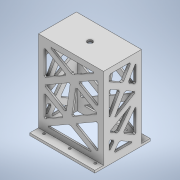
# Autodesk Inventor part: Shroud
Saved by Autodesk Inventor 2020 (Build 240168000, 168)
## iProperties
Created: 2019-08-01
Part Number: Shroud
Material: Generic
Document SubType Name: Modeling
Designer: Alex
Density: 1 g/cm^3
Appearance: Default
Author: Alex
Autodesk Inventor part; units mm, degrees
ref_plane "YZ Plane" through (0, 0, 0) normal (1, 0, 0) x (0, 1, 0)
ref_plane "XZ Plane" through (0, 0, 0) normal (0, 1, 0) x (-1, 0, 0)
ref_plane "XY Plane" through (0, 0, 0) normal (0, 0, 1) x (1, 0, 0)
sketch "Sketch3" plane through (0, 0, 0) normal (0, 1, 0) x (-1, 0, 0)
  line L0 (41.166, -35) -> (-41.166, -35)
  line L1 (-41.166, -35) -> (-41.166, 35)
  line L2 (-41.166, 35) -> (41.166, 35)
  line L3 (41.166, 35) -> (41.166, -35)
  line L4 (38.166, -22) -> (-38.166, -22)
  line L5 (-38.166, -22) -> (-38.166, 22)
  line L6 (-38.166, 22) -> (38.166, 22)
  line L7 (38.166, 22) -> (38.166, -22)
  point P0 (0, 0)
  point P1 (0, -35)
  point P2 (41.166, 0)
  point P3 (-38.166, 0)
  point P4 (0, -22)
  dimension "d7" = 82.332
  dimension "d8" = 70
  dimension "d10" = 13
  dimension "d12" = 3
  constraints: 16 end point, 4 midpoint, 4 parallel, 2 horizontal, 2 horizontal alignment, 2 perpendicular, 2 vertical alignment
  measures "d7" distance of L1.end L2.end
  measures "d8" distance of L0.end L1.end
  measures "d10" distance between parallel lines of L0 L4
  measures "d12" distance between parallel lines of L1 L5
extrude "Extrusion2" add sketch "Sketch3" along normal blind 3
sketch "Sketch4" plane through (0, 3, 0) normal (0, 1, 0) x (1, 0, 0)
  line L0 (41.166, -35) -> (41.166, 35) construction
  line L1 (41.166, 35) -> (-41.166, 35) construction
  line L2 (-41.166, 35) -> (-41.166, -35) construction
  line L3 (-41.166, -35) -> (41.166, -35) construction
  line L4 (38.166, -22) -> (-38.166, -22) construction
  line L5 (-38.166, -22) -> (-38.166, 22) construction
  line L6 (-38.166, 22) -> (38.166, 22) construction
  line L7 (38.166, 22) -> (38.166, -22) construction
  line L8 (-41.166, 35) -> (-41.166, -35) construction
  line L9 (-41.166, 24) -> (-41.166, -24)
  line L10 (41.166, -24) -> (-41.166, -24)
  line L11 (41.166, -24) -> (41.166, 24)
  line L12 (41.166, -35) -> (41.166, 35) construction
  line L13 (-41.166, 24) -> (41.166, 24)
  line L14 (-38.166, 22) -> (38.166, 22) projected
  line L15 (-38.166, -22) -> (38.166, -22)
  line L16 (38.166, -22) -> (38.166, 22)
  line L17 (38.166, 22) -> (-38.166, 22)
  line L18 (-38.166, 22) -> (-38.166, -22)
  point P0 (0, 0)
  point P1 (-41.166, 0)
  point P2 (-38.166, 0)
  dimension "d16" = 2
  constraints: 16 end point, 4 point on line, 2 horizontal, 2 midpoint, 2 parallel, 2 perpendicular, 1 horizontal alignment
  measures "d16" distance between parallel lines of L13 L6
extrude "Extrusion3" add sketch "Sketch4" along normal blind 100
sketch "Sketch5" plane through (0, 103, 0) normal (0, 1, 0) x (1, 0, 0)
  line L0 (-41.166, -24) -> (41.166, -24) projected
  line L1 (41.166, -24) -> (41.166, 24) projected
  line L2 (41.166, 24) -> (-41.166, 24) projected
  line L3 (-41.166, 24) -> (-41.166, -24) projected
  line L4 (38.166, 22) -> (38.166, -22) construction
  line L5 (38.166, -22) -> (-38.166, -22) construction
  line L6 (-38.166, -22) -> (-38.166, 22) construction
  line L7 (-38.166, 22) -> (38.166, 22) construction
  point P0 (0, 0)
extrude "Extrusion4" add sketch "Sketch5" along normal blind 3
sketch "Sketch6" plane through (-41.166, 0, -35) normal (-1, 0, 0) x (0, 0, 1)
  line L0 (0, 0) -> (70, 0) construction
  line L1 (57, 0) -> (13, 0) construction
  arc A0 (39, 0) -> (31, 0) centre (35, 0) ccw
  line L2 (31, 0) -> (39, 0)
  point P0 (35, 0)
  dimension "d22" = 4
  constraints: 2 end point, 2 point on circle, 2 point on line, 1 centre point, 1 coincident, 1 midpoint
  measures "d22" radius of A0
extrude "Extrusion5" cut sketch "Sketch6" against normal up to surface (3 mm away)
sketch "Sketch7" plane through (0, 3, 0) normal (0, 1, 0) x (1, 0, 0)
  line L0 (41.166, -35) -> (41.166, 35) construction
  line L1 (41.166, 35) -> (-41.166, 35) construction
  line L2 (-41.166, -35) -> (41.166, -35) construction
  point P0 (0, 0)
  point P1 (33.834, 27)
  point P2 (1.334, 27)
  point P3 (-31.166, 27)
  point P4 (-31.166, -27)
  point P5 (1.334, -27)
  point P6 (33.834, -27)
  dimension "d25" = 7.332
  dimension "d26" = 39.832
  dimension "d27" = 72.332
  dimension "d28" = 8
  dimension "d29" = 8
  constraints: 4 horizontal alignment, 3 vertical alignment
  measures "d25" distance from line of point (33.834, 27) L0
  measures "d26" distance from line of point (1.334, 27) L0
  measures "d27" distance from line of point (-31.166, 27) L0
  measures "d28" distance from line of L1 point (33.834, 27)
  measures "d29" distance from line of L2 point (33.834, -27)
hole "Hole1" at (33.834, 3, -27) at (1.334, 3, -27) at (-31.166, 3, -27) at (-31.166, 3, 27) at (1.334, 3, 27) at (33.834, 3, 27) direction (0, -1, 0) diameter 3 end through all
sketch "Sketch8" plane through (-41.166, 3, 24) normal (0, 0, 1) x (1, 0, 0)
  line L0 (82.332, 0) -> (0, 0) construction
  line L1 (82.332, 0) -> (82.332, 103) construction
  line L2 (0, 103) -> (82.332, 103) construction
  line L3 (0, 0) -> (0, 103) construction
  line L4 (75.332, 96) -> (75.332, 7) construction
  line L5 (75.332, 7) -> (7, 7) construction
  line L6 (7, 7) -> (7, 96) construction
  line L7 (7, 96) -> (75.332, 96) construction
  line L8 (14.0115, 96) -> (75.332, 60.5966) construction
  line L9 (75.332, 52.5137) -> (7, 91.9652) construction
  line L10 (75.332, 52.5137) -> (7, 13.0622) construction
  line L11 (10.5, 7) -> (75.332, 44.4308) construction
  line L12 (7, 13.0622) -> (10.5, 7) construction
  line L13 (35.9217, 75.2672) -> (7, 58.5692) construction
  line L14 (7, 50.4863) -> (42.9217, 71.2257) construction
  line L15 (7, 50.4863) -> (39.4103, 31.7743) construction
  line L16 (7, 42.4034) -> (32.4103, 27.7328) construction
  line L17 (42.9217, 79.3087) -> (71.832, 96) construction
  line L18 (75.332, 89.9378) -> (49.9217, 75.2672) construction
  line L19 (71.832, 96) -> (75.332, 89.9378) construction
  line L20 (39.4103, 23.6913) -> (75.332, 2.9519) construction
  line L21 (46.4103, 27.7328) -> (75.332, 11.0348) construction
  line L22 (40.3575, 69.7453) -> (35.0516, 34.2907) construction
  line L23 (47.2804, 68.7093) -> (41.9745, 33.2547) construction
  line L24 (40.3575, 69.7453) -> (47.2804, 68.7093) construction
  line L25 (35.0516, 34.2907) -> (41.9745, 33.2547) construction
  line L26 (15.7435, 95) -> (41.1897, 80.3087)
  line L27 (44.6538, 80.3087) -> (70.0999, 95)
  line L28 (69.832, 96) -> (16.0115, 96)
  line L29 (34.1897, 76.2672) -> (8.7321, 90.9652)
  line L30 (7, 60.5692) -> (7, 89.9652)
  line L31 (8.7321, 59.5692) -> (34.1897, 74.2672)
  line L32 (51.6538, 76.2672) -> (73.5999, 88.9378)
  line L33 (75.332, 62.5966) -> (75.332, 87.9378)
  line L34 (51.6538, 74.2672) -> (73.5999, 61.5966)
  line L35 (46.9844, 66.7313) -> (42.2705, 35.2327)
  line L36 (43.7065, 34.2547) -> (73.5999, 51.5137)
  line L37 (73.5999, 53.5137) -> (49.0125, 67.7093)
  line L38 (8.7321, 49.4863) -> (33.3195, 35.2907)
  line L39 (35.3476, 36.2687) -> (40.0615, 67.7673)
  line L40 (8.7321, 51.4863) -> (38.6255, 68.7453)
  line L41 (7, 40.4034) -> (7, 15.0622)
  line L42 (8.7321, 14.0622) -> (30.6782, 26.7328)
  line L43 (30.6782, 28.7328) -> (8.7321, 41.4034)
  line L44 (12.2321, 8) -> (37.6782, 22.6913)
  line L45 (41.1423, 22.6913) -> (66.5885, 8)
  line L46 (66.3205, 7) -> (12.5, 7)
  line L47 (48.1423, 28.7328) -> (73.5999, 43.4308)
  line L48 (75.332, 42.4308) -> (75.332, 13.0348)
  line L49 (48.1423, 26.7328) -> (73.5999, 12.0348)
  line L50 (8.7321, 90.9652) -> (7, 89.9652)
  line L51 (7, 60.5692) -> (8.7321, 59.5692)
  line L52 (7, 60.5692) -> (8.7321, 59.5692)
  line L53 (34.1897, 74.2672) -> (34.1897, 76.2672)
  line L54 (15.7435, 95) -> (16.0115, 96)
  line L55 (70.0999, 95) -> (69.832, 96)
  line L56 (69.832, 96) -> (70.0999, 95)
  line L57 (41.1897, 80.3087) -> (44.6538, 80.3087)
  line L58 (51.6538, 74.2672) -> (51.6538, 76.2672)
  line L59 (73.5999, 88.9378) -> (75.332, 87.9378)
  line L60 (73.5999, 61.5966) -> (75.332, 62.5966)
  line L61 (49.0125, 67.7093) -> (46.9844, 66.7313)
  line L62 (42.2705, 35.2327) -> (43.7065, 34.2547)
  line L63 (73.5999, 53.5137) -> (73.5999, 51.5137)
  line L64 (8.7321, 41.4034) -> (7, 40.4034)
  line L65 (8.7321, 41.4034) -> (7, 40.4034)
  line L66 (8.7321, 14.0622) -> (7, 15.0622)
  line L67 (30.6782, 26.7328) -> (30.6782, 28.7328)
  line L68 (12.2321, 8) -> (12.5, 7)
  line L69 (66.5885, 8) -> (66.3205, 7)
  line L70 (37.6782, 22.6913) -> (41.1423, 22.6913)
  line L71 (48.1423, 28.7328) -> (48.1423, 26.7328)
  line L72 (73.5999, 43.4308) -> (75.332, 42.4308)
  line L73 (73.5999, 12.0348) -> (75.332, 13.0348)
  line L74 (8.7321, 49.4863) -> (8.7321, 51.4863)
  line L75 (8.7321, 49.4863) -> (8.7321, 51.4863)
  line L76 (38.6255, 68.7453) -> (40.0615, 67.7673)
  line L77 (33.3195, 35.2907) -> (35.3476, 36.2687)
  point P0 (41.166, -3)
  point P1 (68.3205, 7)
  dimension "d37" = 7
  dimension "d38" = 30
  dimension "d39" = 60
  dimension "d40" = 7
  dimension "d41" = 7
  dimension "d42" = 7
  dimension "d43" = 7
  dimension "d44" = 60
  dimension "d45" = 60
  dimension "d46" = 7
  dimension "d49" = 2
  dimension "d50" = 2
  dimension "d51" = 2
  dimension "d52" = 2
  dimension "d53" = 2
  dimension "d54" = 2
  dimension "d55" = 2
  dimension "d56" = 2
  dimension "d57" = 2
  dimension "d58" = 2
  dimension "d59" = 2
  dimension "d60" = 2
  dimension "d61" = 2
  dimension "d62" = 2
  dimension "d63" = 2
  dimension "d64" = 2
  dimension "d65" = 2
  dimension "d66" = 2
  dimension "d67" = 2
  dimension "d68" = 2
  dimension "d69" = 2
  dimension "d70" = 2
  dimension "d71" = 2
  dimension "d72" = 2
  dimension "d73" = 2
  dimension "d74" = 2
  dimension "d75" = 2
  dimension "d76" = 2
  dimension "d77" = 2
  dimension "d78" = 2
  dimension "d79" = 2
  dimension "d80" = 2
  dimension "d81" = 2
  dimension "d82" = 2
  dimension "d83" = 2
  dimension "d84" = 2
  dimension "d85" = 2
  dimension "d86" = 2
  dimension "d87" = 2
  dimension "d88" = 2
  dimension "d89" = 2
  dimension "d90" = 2
  dimension "d91" = 2
  dimension "d92" = 2
  dimension "d93" = 2
  dimension "d94" = 2
  dimension "d95" = 2
  dimension "d96" = 2
  dimension "d97" = 2
  dimension "d98" = 2
  dimension "d99" = 2
  dimension "d100" = 2
  dimension "d101" = 2
  dimension "d102" = 2
  constraints: 148 end point, 91 point on line, 20 collinear, 9 parallel, 7 perpendicular, 3 other
  measures "d37" distance between parallel lines of L2 L7
  measures "d38" angle of L11 L5
  measures "d39" angle of L10 L9
  measures "d40" distance between parallel lines of L11 L10
  measures "d41" distance between parallel lines of L8 L9
  measures "d42" distance between parallel lines of L13 L14
  measures "d43" distance between parallel lines of L15 L16
  measures "d44" angle of L10 L16
  measures "d45" angle of L14 L15
  measures "d46" distance between parallel lines of L23 L22
  measures "d49" distance of L29.end L9.end
  measures "d50" distance of L30.end L9.end
  measures "d51" distance of L51.start L13.end
  measures "d52" distance of L51.end L13.end
  measures "d53" distance of L30.start point (7, 58.569)
  measures "d54" distance of L31.start point (7, 58.569)
  measures "d55" distance of L31.end L13.start
  measures "d56" distance of L29.start L13.start
  measures "d57" distance of L26.start L8.start
  measures "d58" distance of L28.end L8.start
  measures "d59" distance of L55.start L17.end
  measures "d60" distance of L55.end L17.end
  measures "d61" distance of L28.start point (71.832, 96)
  measures "d62" distance of L27.end point (71.832, 96)
  measures "d63" distance of L26.end L17.start
  measures "d64" distance of L27.start L17.start
  measures "d65" distance of L34.start L18.end
  measures "d66" distance of L32.start L18.end
  measures "d67" distance of L32.end L18.start
  measures "d68" distance of L33.end L18.start
  measures "d69" distance of L34.end L8.end
  measures "d70" distance of L33.start L8.end
  measures "d71" distance of L37.end L23.start
  measures "d72" distance of L35.start L23.start
  measures "d73" distance of L35.end L23.end
  measures "d74" distance of L36.start L23.end
  measures "d75" distance of L37.start L9.start
  measures "d76" distance of L36.end L9.start
  measures "d77" distance of L64.start L16.start
  measures "d78" distance of L64.end L16.start
  measures "d79" distance of L43.end point (7, 42.403)
  measures "d80" distance of L41.start point (7, 42.403)
  measures "d81" distance of L42.start L10.end
  measures "d82" distance of L41.end L10.end
  measures "d83" distance of L42.end L16.end
  measures "d84" distance of L43.start L16.end
  measures "d85" distance of L44.start L11.start
  measures "d86" distance of L46.end L11.start
  measures "d87" distance of L45.end point (68.321, 7)
  measures "d88" distance of L46.start point (68.321, 7)
  measures "d89" distance of L44.end L20.start
  measures "d90" distance of L45.start L20.start
  measures "d91" distance of L47.start L21.start
  measures "d92" distance of L49.start L21.start
  measures "d93" distance of L47.end L11.end
  measures "d94" distance of L48.start L11.end
  measures "d95" distance of L49.end L21.end
  measures "d96" distance of L48.end L21.end
  measures "d97" distance of L74.start L14.start
  measures "d98" distance of L74.end L14.start
  measures "d99" distance of L38.start point (7, 50.486)
  measures "d100" distance of L40.start point (7, 50.486)
  measures "d101" distance of L40.end L22.start
  measures "d102" distance of L39.end L22.start
extrude "Extrusion6" cut sketch "Sketch8" against normal through all
sketch "Sketch9" plane through (-41.166, 3, 24) normal (-1, 0, 0) x (0, 0, 1)
  arc A0 (-20, -3) -> (-28, -3) centre (-24, -3) ccw construction
  line L0 (-20, -3) -> (11, -3) construction
  line L1 (11, -3) -> (11, 0) construction
  line L2 (0, 0) -> (11, 0) construction
  line L3 (0, 0) -> (0, 103) construction
  line L4 (-48, 103) -> (0, 103) construction
  line L5 (-48, 0) -> (-48, 103) construction
  line L6 (-59, 0) -> (-48, 0) construction
  line L7 (-59, -3) -> (-59, 0) construction
  line L8 (-59, -3) -> (-28, -3) construction
  line L9 (-41, 96) -> (-7, 96) construction
  line L10 (-7, 96) -> (-7, 7) construction
  line L11 (-7, 7) -> (-41, 7) construction
  line L12 (-41, 7) -> (-41, 96) construction
  line L13 (-41, 13.0622) -> (-7, 32.6921) construction
  line L14 (-37.5, 7) -> (-7, 24.6092) construction
  line L15 (-7, 32.6921) -> (-41, 52.322) construction
  line L16 (-7, 88.1177) -> (-41, 68.4878) construction
  line L17 (-41, 60.4049) -> (-7, 40.775) construction
  line L18 (-41, 60.4049) -> (-7, 80.0348) construction
  line L19 (-41, 92.5) -> (-30.6024, 74.4909) construction
  line L20 (-24.5402, 77.9909) -> (-34.9378, 96) construction
  line L21 (-41, 92.5) -> (-34.9378, 96) construction
  line L22 (-41, 13.0622) -> (-37.5, 7) construction
  line L23 (-27.1024, 68.4287) -> (-13.2048, 44.3573) construction
  line L24 (-21.0402, 71.9287) -> (-7, 47.6103) construction
  line L25 (-12.6013, 7) -> (-41, 44.8898) construction
  line L26 (-7, 11.1982) -> (-35.3987, 49.0881) construction
  line L27 (-12.6013, 7) -> (-7, 11.1982) construction
  line L28 (-41, 44.8898) -> (-35.3987, 49.0881) construction
  line L29 (-33.9378, 94.2679) -> (-25.5402, 79.7229)
  line L30 (-22.8082, 78.9909) -> (-7, 88.1177)
  line L31 (-7, 88.1177) -> (-7, 94)
  line L32 (-9, 96) -> (-32.9378, 96)
  line L33 (-40, 90.7679) -> (-31.6024, 76.2229)
  line L34 (-32.3345, 73.4909) -> (-39.2679, 69.4878)
  line L35 (-41, 90.5) -> (-41, 70.4878)
  line L36 (-19.3082, 72.9287) -> (-8.7321, 79.0348)
  line L37 (-20.0402, 70.1966) -> (-8, 49.3423)
  line L38 (-7, 49.6103) -> (-7, 78.0348)
  line L39 (-26.1024, 66.6966) -> (-14.2048, 46.0894)
  line L40 (-39.2679, 61.4049) -> (-28.8345, 67.4287)
  line L41 (-39.2679, 59.4049) -> (-14.9369, 45.3573)
  line L42 (-34.1992, 47.4877) -> (-19.4436, 27.8007)
  line L43 (-8.7321, 31.6921) -> (-16.5121, 27.2003)
  line L44 (-33.6666, 48.0881) -> (-8.7321, 33.6921)
  line L45 (-39.8005, 43.2895) -> (-25.5494, 24.2755)
  line L46 (-26.082, 21.6751) -> (-39.2679, 14.0622)
  line L47 (-41, 15.0622) -> (-41, 42.8898)
  line L48 (-35.7679, 8) -> (-21.8535, 16.0335)
  line L49 (-13.8008, 8.6004) -> (-18.922, 15.4331)
  line L50 (-14.6013, 7) -> (-35.5, 7)
  line L51 (-8.1995, 12.7986) -> (-12.8162, 18.9583)
  line L52 (-8.7321, 23.6092) -> (-12.2837, 21.5587)
  line L53 (-7, 22.6092) -> (-7, 13.1982)
  line L54 (-41, 70.4878) -> (-39.2679, 69.4878)
  line L55 (-32.3345, 73.4909) -> (-31.6024, 76.2229)
  line L56 (-41, 90.5) -> (-40, 90.7679)
  line L57 (-33.9378, 94.2679) -> (-32.9378, 96)
  line L58 (-22.8082, 78.9909) -> (-25.5402, 79.7229)
  line L59 (-9, 96) -> (-7, 94)
  line L60 (-20.0402, 70.1966) -> (-19.3082, 72.9287)
  line L61 (-7, 78.0348) -> (-8.7321, 79.0348)
  line L62 (-8, 49.3423) -> (-7, 49.6103)
  line L63 (-14.2048, 46.0894) -> (-14.9369, 45.3573)
  line L64 (-39.2679, 59.4049) -> (-39.2679, 61.4049)
  line L65 (-28.8345, 67.4287) -> (-26.1024, 66.6966)
  line L66 (-34.1992, 47.4877) -> (-33.6666, 48.0881)
  line L67 (-19.4436, 27.8007) -> (-16.5121, 27.2003)
  line L68 (-8.7321, 33.6921) -> (-8.7321, 31.6921)
  line L69 (-41, 42.8898) -> (-39.8005, 43.2895)
  line L70 (-41, 15.0622) -> (-39.2679, 14.0622)
  line L71 (-26.082, 21.6751) -> (-25.5494, 24.2755)
  line L72 (-35.7679, 8) -> (-35.5, 7)
  line L73 (-21.8535, 16.0335) -> (-18.922, 15.4331)
  line L74 (-14.6013, 7) -> (-13.8008, 8.6004)
  line L75 (-12.8162, 18.9583) -> (-12.2837, 21.5587)
  line L76 (-8.7321, 23.6092) -> (-7, 22.6092)
  line L77 (-8.1995, 12.7986) -> (-7, 13.1982)
  point P0 (-24, -3)
  point P1 (-18.2441, 26.2003)
  point P2 (-24.3499, 22.6751)
  point P3 (-20.1215, 17.0335)
  point P4 (-14.0157, 20.5587)
  dimension "d105" = 7
  dimension "d106" = 7
  dimension "d107" = 7
  dimension "d108" = 7
  dimension "d109" = 30
  dimension "d110" = 60
  dimension "d111" = 7
  dimension "d112" = 7
  dimension "d113" = 7
  dimension "d114" = 60
  dimension "d115" = 7
  dimension "d116" = 7
  dimension "d117" = 2
  dimension "d118" = 2
  dimension "d119" = 2
  dimension "d120" = 2
  dimension "d121" = 2
  dimension "d122" = 2
  dimension "d123" = 2
  dimension "d124" = 2
  dimension "d125" = 2
  dimension "d126" = 2
  dimension "d127" = 2
  dimension "d128" = 2
  dimension "d129" = 2
  dimension "d130" = 2
  dimension "d131" = 2
  dimension "d132" = 2
  dimension "d133" = 2
  dimension "d134" = 2
  dimension "d135" = 2
  dimension "d136" = 2
  dimension "d137" = 2
  dimension "d138" = 2
  dimension "d139" = 2
  dimension "d140" = 2
  dimension "d141" = 2
  dimension "d142" = 2
  dimension "d143" = 2
  dimension "d144" = 2
  dimension "d145" = 2
  dimension "d146" = 2
  dimension "d147" = 2
  dimension "d148" = 2
  dimension "d149" = 2
  dimension "d150" = 2
  dimension "d151" = 2
  dimension "d152" = 2
  dimension "d153" = 2
  dimension "d154" = 2
  dimension "d155" = 2
  dimension "d156" = 2
  dimension "d157" = 2
  dimension "d158" = 2
  dimension "d159" = 2
  dimension "d160" = 2
  dimension "d161" = 2
  dimension "d162" = 2
  dimension "d163" = 2
  dimension "d164" = 2
  constraints: 136 end point, 79 point on line, 9 collinear, 9 perpendicular, 7 parallel, 3 vertical, 2 horizontal, 10 other
  measures "d105" distance between parallel lines of L5 L12
  measures "d106" distance between parallel lines of L4 L9
  measures "d108" distance from line of L11 L5.start
  measures "d109" angle of L11 L14
  measures "d110" angle of L15 L13
  measures "d111" distance between parallel lines of L14 L13
  measures "d112" distance between parallel lines of L15 L17
  measures "d113" distance between parallel lines of L18 L16
  measures "d114" angle of L18 L17
  measures "d115" distance between parallel lines of L20 L19
  measures "d116" distance between parallel lines of L26 L25
  measures "d117" distance of L35.end L16.end
  measures "d118" distance of L34.end L16.end
  measures "d119" distance of L34.start L19.end
  measures "d120" distance of L33.end L19.end
  measures "d121" distance of L35.start L19.start
  measures "d122" distance of L33.start L19.start
  measures "d123" distance of L29.start L20.end
  measures "d124" distance of L32.end L20.end
  measures "d125" distance of L30.start L20.start
  measures "d126" distance of L29.end L20.start
  measures "d127" distance of L32.start L9.end
  measures "d128" distance of L31.end L9.end
  measures "d129" distance of L37.start L24.start
  measures "d130" distance of L36.start L24.start
  measures "d131" distance of L38.end L18.end
  measures "d132" distance of L36.end L18.end
  measures "d133" distance of L37.end L24.end
  measures "d134" distance of L38.start L24.end
  measures "d135" distance of L39.end L23.end
  measures "d136" distance of L41.end L23.end
  measures "d137" distance of L41.start L17.start
  measures "d138" distance of L40.start L17.start
  measures "d139" distance of L40.end L23.start
  measures "d140" distance of L39.start L23.start
  measures "d141" distance of L42.start L26.end
  measures "d142" distance of L44.start L26.end
  measures "d143" distance of L42.end point (-18.244, 26.2)
  measures "d144" distance of L43.end point (-18.244, 26.2)
  measures "d145" distance of L44.end point (-7, 32.692)
  measures "d146" distance of L43.start point (-7, 32.692)
  measures "d147" distance of L47.end L25.end
  measures "d148" distance of L45.start L25.end
  measures "d149" distance of L47.start point (-41, 13.062)
  measures "d150" distance of L46.end point (-41, 13.062)
  measures "d151" distance of L46.start point (-24.35, 22.675)
  measures "d152" distance of L45.end point (-24.35, 22.675)
  measures "d153" distance of L48.start L14.start
  measures "d154" distance of L50.end L14.start
  measures "d155" distance of L48.end point (-20.121, 17.033)
  measures "d156" distance of L49.end point (-20.121, 17.033)
  measures "d157" distance of L50.start L25.start
  measures "d158" distance of L49.start L25.start
  measures "d159" distance of L51.end point (-14.016, 20.559)
  measures "d160" distance of L52.end point (-14.016, 20.559)
  measures "d161" distance of L52.start L14.end
  measures "d162" distance of L53.start L14.end
  measures "d163" distance of L51.start point (-7, 11.198)
  measures "d164" distance of L53.end point (-7, 11.198)
extrude "Extrusion7" cut sketch "Sketch9" against normal through all
sketch "Sketch10" plane through (0, 106, 0) normal (0, 1, 0) x (1, 0, 0)
  point P0 (0, 0)
  point P1 (0, 0)
  constraints: 1 coincident
hole "Hole2" at (0, 106, 0) direction (0, -1, 0) diameter 6.5 depth 10
equation "\"d40\" = d37"
equation "\"d41\" = d37"
equation "\"d42\" = d37"
equation "\"d43\" = d37"
equation "\"d46\" = d37"
equation "\"d50\" = d49"
equation "\"d52\" = d51"
equation "\"d54\" = d53"
equation "\"d55\" = d53"
equation "\"d56\" = d55"
equation "\"d58\" = d57"
equation "\"d60\" = d59"
equation "\"d62\" = d61"
equation "\"d64\" = d63"
equation "\"d66\" = d65"
equation "\"d68\" = d67"
equation "\"d70\" = d69"
equation "\"d72\" = d71"
equation "\"d74\" = d73"
equation "\"d76\" = d75"
equation "\"d78\" = d77"
equation "\"d80\" = d79"
equation "\"d82\" = d81"
equation "\"d84\" = d83"
equation "\"d86\" = d85"
equation "\"d88\" = d87"
equation "\"d90\" = d89"
equation "\"d92\" = d91"
equation "\"d94\" = d93"
equation "\"d96\" = d95"
equation "\"d98\" = d97"
equation "\"d100\" = d99"
equation "\"d102\" = d101"
equation "\"d105\" = d37"
equation "\"d106\" = d37"
equation "\"d107\" = d37"
equation "\"d108\" = d37"
body "Solid2"
